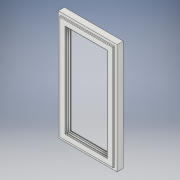
# Autodesk Inventor part: Окно-01
Saved by Autodesk Inventor 2019 (Build 230136000, 136)
## iProperties
Created: 2018-09-18
Part Number: Окно-01
Material: Пластик АБС
Document SubType Name: Modeling
Designer: Андреев Н.Л.
Density: 1.06 g/cm^3
Appearance: Гладкий — белый
ДЛИНА: 800,000 мм
ШИРИНА: 1500,000 мм
ТОЛЩВЫС: 105,000 мм
Author: Андреев Н.Л.
Autodesk Inventor part; units mm, degrees
ref_plane "YZ Plane" through (0, 0, 0) normal (1, 0, 0) x (0, 1, 0)
ref_plane "XZ Plane" through (0, 0, 0) normal (0, 1, 0) x (-1, 0, 0)
ref_plane "XY Plane" through (0, 0, 0) normal (0, 0, 1) x (1, 0, 0)
sketch "Эскиз2" plane through (0, 0, 0) normal (0, 1, 0) x (-1, 0, 0)
  line L0 (0.1799, 0.0907) -> (0.1799, 84.0907)
  line L1 (0.1799, 0.0907) -> (-61.0397, 0.0907)
  arc A0 (-65.7382, 3.3806) -> (-61.0397, 0.0907) centre (-61.0397, 5.0907) ccw
  line L2 (-65.7382, 3.3806) -> (-71.8201, 20.0907)
  line L3 (-71.8201, 20.0907) -> (-44.8201, 20.0907)
  line L4 (-44.8201, 20.0907) -> (-44.8201, 84.0907)
  line L5 (-44.8201, 84.0907) -> (0.1799, 84.0907)
  line L6 (-63.38, 20.0907) -> (-108.2723, 20.0907)
  arc A1 (-116.2117, 25.7655) -> (-108.2723, 20.0907) centre (-108.2723, 28.4819) ccw
  line L7 (-116.2117, 25.7655) -> (-119.8201, 36.3123)
  line L8 (-119.8201, 36.3123) -> (-119.8201, 40.5963)
  line L9 (-119.8201, 40.5963) -> (-99.6925, 40.5963)
  line L10 (-99.6925, 40.5963) -> (-99.6925, 88.5963)
  line L11 (-99.6925, 88.5963) -> (-119.8201, 88.5963)
  line L12 (-119.8201, 88.5963) -> (-119.8201, 91.7931)
  line L13 (-119.8201, 91.7931) -> (-117.1981, 101.1835)
  arc A2 (-111.7107, 105.0907) -> (-117.1981, 101.1835) centre (-111.7107, 99.2838) ccw
  line L14 (-111.7107, 105.0907) -> (-42.8025, 105.0907)
  arc A3 (-35.8201, 98.1083) -> (-42.8025, 105.0907) centre (-42.8025, 98.1083) ccw
  line L15 (-35.8201, 98.1083) -> (-35.8201, 84.0907)
  line L16 (-35.8201, 84.0907) -> (-57.8942, 84.0907)
  line L17 (-57.8942, 84.0907) -> (-57.8942, 43.1736)
  line L18 (-57.8942, 43.1736) -> (-63.38, 43.1736)
  line L19 (-63.38, 43.1736) -> (-63.38, 20.0907)
  dimension "d14" = 84
  dimension "d15" = 72
  dimension "d16" = 5
  dimension "d17" = 110
  dimension "d18" = 20
  dimension "d19" = 45
  dimension "d20" = 120
  dimension "d21" = 48
  dimension "d22" = 36
  dimension "ТОЛЩВЫС" = 105
  constraints: 40 end point, 10 perpendicular, 8 point on circle, 7 tangent, 4 centre point, 2 collinear, 2 point on line
  measures "d14" distance of L1.start L0.end
  measures "d15" distance from line of L0 L3.start
  measures "d16" radius of A0
  measures "d17" angle of L1 L2
  measures "d18" distance between parallel lines of L3 L1
  measures "d19" distance between parallel lines of L0 L4
  measures "d20" distance between parallel lines of L8 L0
  measures "d21" distance between parallel lines of L11 L9
  measures "d22" distance between parallel lines of L15 L0
  measures "ТОЛЩВЫС" distance between parallel lines of L14 L1
sketch "Эскиз1" plane through (0, 0, 0) normal (0, 0, 1) x (1, 0, 0)
  line L0 (0, 0) -> (800, 0)
  line L1 (800, 0) -> (800, 1500)
  line L2 (800, 1500) -> (0, 1500)
  line L3 (0, 1500) -> (0, 0)
  dimension "ДЛИНА" = 800
  dimension "ШИРИНА" = 1500
  constraints: 8 end point, 2 parallel, 1 horizontal, 1 perpendicular
  measures "ДЛИНА" distance of L2.end L1.end
  measures "ШИРИНА" distance of L1.end L0.end
sweep "Сдвиг1" add profiles "Эскиз2" path "Эскиз1" path curves L3 L2 L1 L0 contours L1 A0 L2 L3 L4 L5 L0
sweep "Сдвиг2" add profiles "Эскиз2" path "Эскиз1" separate body path curves L3 L2 L1 L0 contours L5 L16 L17 L18 L19 L3 L6 A1 L7 L8 L9 L10 L11 L12 L13 A2 L14 A3 L15
sketch "Эскиз3" plane through (99.6925, 99.6925, 40.5963) normal (0, 1, 0) x (1, 0, 0)
  line L0 (0, -48) -> (600.615, -48)
  line L1 (600.615, -48) -> (600.615, -43)
  line L2 (600.615, -43) -> (0, -43)
  line L3 (0, -43) -> (0, -48)
  line L4 (600.615, -48) -> (600.615, 0) construction
  line L5 (600.615, 0) -> (0, 0) construction
  line L6 (0, -48) -> (0, 0) construction
  line L7 (600.615, -48) -> (0, -48) construction
  point P0 (-99.6925, 40.5963)
  dimension "ТолщСтекла" = 5
  constraints: 8 end point, 3 collinear, 2 parallel, 1 horizontal, 1 perpendicular
  measures "ТолщСтекла" distance of L1.end L0.end
extrude "Выдавливание1" add sketch "Эскиз3" along normal up to next separate body
pattern_linear "Прямоуг.массив1" count 3 spacing 21.5 along (0, 0, -1) of "Выдавливание1" bodies 3
